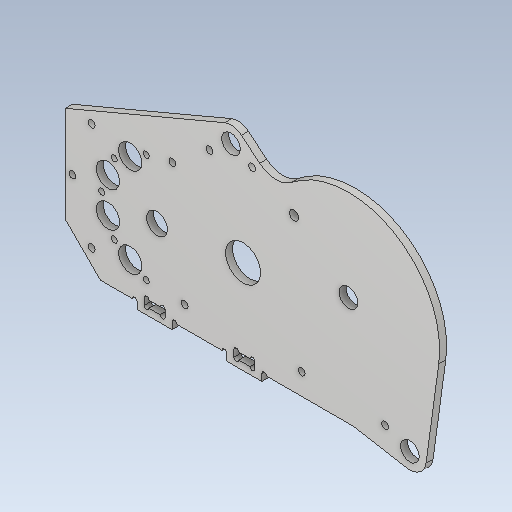
# Autodesk Inventor part: アーム真ん中フレーム
Saved by Autodesk Inventor 2020 (Build 240168000, 168)
## iProperties
Created: 2019-12-03
Part Number: アーム真ん中フレーム
Material: アルミニウム 2014-T4
Document SubType Name: Modeling
Designer: tanjihayato
Density: 2.8 g/cm^3
Appearance: サテン
Mass: 94.056 g
Surface Area: 251.98 cm^2
Volume: 33.5914 cm^3
Author: tanjihayato
Autodesk Inventor part; units mm, degrees
note: some values were not read from the file. Chosen so that the rebuilt part matches the saved one: sketch regions of "押し出し1".
ref_plane "YZ Plane" through (0, 0, 0) normal (1, 0, 0) x (0, 1, 0)
ref_plane "XZ Plane" through (0, 0, 0) normal (0, 1, 0) x (-1, 0, 0)
ref_plane "XY Plane" through (0, 0, 0) normal (0, 0, 1) x (1, 0, 0)
sketch "スケッチ1" plane through (0, 0, 0) normal (0, 0, 1) x (1, 0, 0)
  line L0 (-170.6512, -31.4118) -> (202.8656, -31.4118) construction
  circle A0 centre (-14, -17.4118) radius 14 construction
  circle A1 centre (14, -17.4118) radius 14 construction
  circle A2 centre (-28.0204, 0.0121) radius 20.05 construction
  circle A3 centre (-28.0204, 0.0121) radius 5.05 construction
  circle A4 centre (8.8763, 3.8907) radius 32.05 construction
  circle A5 centre (8.8763, 3.8907) radius 10.1 construction
  circle A6 centre (54.047, 13.5882) radius 36.1 construction
  line L1 (-170.915, -81.4118) -> (490.0044, -81.4118)
  circle A7 centre (-28.0204, 0.0121) radius 22.342 construction
  circle A8 centre (-39.4931, 19.1835) radius 14 construction
  circle A9 centre (-49.0547, 7.5438) radius 14 construction
  circle A10 centre (-49.0547, -7.5196) radius 14 construction
  circle A11 centre (-39.4931, -19.1593) radius 14 construction
  circle A12 centre (8.8763, 3.8907) radius 33.05 construction
  circle A13 centre (54.047, 13.5882) radius 38.1 construction
  line L2 (-11.5565, -29.1593) -> (4.2969, -29.1593) construction
  line L3 (-67.2952, 44.8622) -> (-67.2952, -57.3934) construction
  line L4 (-149.4523, -1.6098) -> (-132.6633, -31.6026)
  line L5 (-132.7701, -31.4118) -> (-132.7701, 74.0456)
  circle A14 centre (-11.4931, -19.1593) radius 14 construction
  line L6 (-197.2268, -33.1593) -> (179.6604, -33.1593) construction
  circle A15 centre (54.047, 13.5882) radius 4.025
  circle A16 centre (54.047, 13.5882) radius 6
  circle A17 centre (-39.4931, 19.1835) radius 5
  circle A18 centre (-49.0547, 7.5438) radius 5
  circle A19 centre (-49.0547, -7.5196) radius 5
  circle A20 centre (-39.4931, -19.1593) radius 5
  circle A21 centre (-39.4931, 19.1835) radius 8 construction
  circle A22 centre (-49.0547, 7.5438) radius 8 construction
  circle A23 centre (-49.0547, -7.5196) radius 8 construction
  circle A24 centre (-39.4931, -19.1593) radius 8 construction
  circle A25 centre (-28.0204, 0.0121) radius 4.5
  circle A26 centre (8.8763, 3.8907) radius 7.5
  line L7 (-17.5497, 32.3149) -> (-46.3578, 15.0755) construction
  line L8 (-46.3578, 15.0755) -> (-51.7515, 0.0121) construction
  line L9 (-51.7515, 0.0121) -> (-46.3578, -15.0513) construction
  line L10 (-46.3578, -15.0513) -> (-37.9391, -20.0892) construction
  circle A27 centre (-32.6283, 23.2915) radius 1.3
  circle A28 centre (-46.3578, 15.0755) radius 1.3
  circle A29 centre (-51.7515, 0.0121) radius 1.3
  circle A30 centre (-46.3578, -15.0513) radius 1.3
  circle A31 centre (-32.6283, -23.2673) radius 1.3
  line L11 (-67.2952, 23.1796) -> (-67.2952, -18.1327)
  arc A32 (79.2003, -37.212) -> (87.3507, -31.2711) centre (80.4159, -30.3183) ccw
  arc A33 (8.1864, 50.8943) -> (0.9804, 51.9708) centre (3.7003, 45.5208) ccw
  line L12 (-52.2685, -33.1593) -> (56.2168, -33.1593)
  line L13 (56.2168, -33.1593) -> (79.2003, -37.212)
  arc A34 (92.7831, 8.2659) -> (29.742, 44.2162) centre (54.047, 13.5882) ccw
  line L14 (87.3507, -31.2711) -> (92.7831, 8.2659)
  line L15 (0.9804, 51.9708) -> (-67.2952, 23.1796)
  circle A35 centre (34.0114, -24.0061) radius 4.5 construction
  circle A36 centre (34.0114, -24.0061) radius 1.5
  circle A37 centre (-21.4477, 26.0369) radius 4.5 construction
  circle A38 centre (-21.4477, 26.0369) radius 1.5
  circle A39 centre (-56.0504, 23.0377) radius 1.5
  circle A40 centre (-56.0504, 23.0377) radius 3 construction
  circle A41 centre (-56.0504, 23.0377) radius 4.5 construction
  circle A42 centre (-64.2952, 0.0121) radius 1.5
  circle A43 centre (-64.2952, 0.0121) radius 3 construction
  circle A44 centre (-64.2952, 0.0121) radius 4.3311 construction
  line L16 (54.047, 13.5882) -> (103.0278, 23.6322)
  line L17 (103.0278, 23.6322) -> (59.4403, 12.4461)
  line L18 (59.4403, 12.4461) -> (30.7326, 32.4678)
  line L19 (30.7326, 32.4678) -> (54.047, 13.5882)
  line L20 (103.0278, 23.6322) -> (519.5307, 130.5215)
  line L21 (-183.2789, 162.2213) -> (-183.2789, -125.2315)
  line L22 (516.7211, 155.5913) -> (516.7211, -155.5644)
  circle A45 centre (103.0278, 23.6322) radius 7.25
  arc A46 (101.805, 33.809) -> (106.8568, 14.1242) centre (103.0278, 23.6322) ccw
  line L23 (141.7723, 33.5754) -> (440.8907, 56.5571) construction
  line L24 (241.9124, 41.2693) -> (202.3713, 99.0317) construction
  circle A47 centre (3.7003, 45.5208) radius 4
  circle A48 centre (127.2431, 29.8467) radius 2
  circle A49 centre (141.7723, 33.5754) radius 2
  arc A50 (143.6401, 28.9373) -> (141.1758, 38.5397) centre (141.7723, 33.5754) ccw
  line L25 (143.6401, 28.9373) -> (106.8568, 14.1242)
  line L26 (141.1758, 38.5397) -> (101.805, 33.809)
  circle A51 centre (30.7326, 32.4678) radius 2
  circle A52 centre (-16.1798, -24.0771) radius 4.5 construction
  circle A53 centre (-16.1798, -24.0771) radius 1.5
  line L27 (-67.2952, -18.1327) -> (-52.2685, -33.1593)
  circle A54 centre (-56.0504, -23.0135) radius 1.5
  circle A55 centre (-56.0504, -23.0135) radius 3 construction
  circle A56 centre (30.7326, 32.4678) radius 4
  arc A57 (55.034, 16.9462) -> (53.2318, 10.1845) centre (54.047, 13.5882) ccw
  line L28 (99.9171, 22.9943) -> (104.0308, 26.6451) construction
  line L29 (104.0308, 26.6451) -> (105.1356, 21.2572) construction
  line L30 (105.1356, 21.2572) -> (99.9171, 22.9943) construction
  circle A58 centre (105.1356, 21.2572) radius 1.5
  circle A59 centre (104.0308, 26.6451) radius 1.5
  circle A60 centre (99.9171, 22.9943) radius 1.5
  circle A61 centre (103.0278, 23.6322) radius 6
  arc A62 (106.7324, 15.9819) -> (96.5933, 29.1862) centre (103.0278, 23.6322) ccw
  arc A63 (55.034, 16.9462) -> (96.5933, 29.1862) centre (66.3134, 55.3229) ccw
  arc A64 (53.2318, 10.1845) -> (106.7324, 15.9819) centre (71.8656, 87.9841) ccw
  circle A65 centre (54.047, 13.5882) radius 8.5
  line L31 (101.3203, 31.9589) -> (52.3395, 21.9149)
  line L32 (55.7545, 5.2615) -> (104.7353, 15.3054)
  circle A66 centre (12.7384, 41.2415) radius 3 construction
  circle A67 centre (12.7384, 41.2415) radius 4.5 construction
  circle A68 centre (12.7384, 41.2415) radius 1.5
  circle A69 centre (80.4159, -30.3183) radius 4
  circle A70 centre (69.7531, -26.0108) radius 1.5
  circle A71 centre (69.7531, -26.0108) radius 4.5 construction
  circle A72 centre (-56.0504, -23.0135) radius 4.5 construction
  line L33 (8.1864, 50.8943) -> (15.9809, 44.3871)
  arc A73 (15.9809, 44.3871) -> (29.742, 44.2162) centre (22.9664, 52.7545) ccw
  circle A74 centre (-5.4761, 38.5895) radius 1.5
  circle A75 centre (-5.4761, 38.5895) radius 4.5 construction
  circle A76 centre (54.047, 13.5882) radius 50 construction
  circle A77 centre (3.7003, 45.5208) radius 2
  circle A78 centre (80.4159, -30.3183) radius 2
  point P0 (0, 0)
  point P1 (0, 0)
  point P2 (-49.0547, 7.5438)
  point P3 (-49.0547, -7.5196)
  dimension "d89" = 100
  dimension "d0" = 40.1
  dimension "d1" = 10.1
  dimension "d2" = 64.1
  dimension "d3" = 20.2
  dimension "d4" = 72.2
  dimension "d5" = 95
  dimension "d6" = 44.684
  dimension "d7" = 28
  dimension "d8" = 28
  dimension "d9" = 28
  dimension "d10" = 28
  dimension "d11" = 1
  dimension "d12" = 2
  dimension "d13" = 4
  dimension "d14" = 8.05
  dimension "d15" = 12
  dimension "d16" = 10
  dimension "d17" = 10
  dimension "d18" = 10
  dimension "d19" = 10
  dimension "d20" = 3
  dimension "d21" = 3
  dimension "d22" = 3
  dimension "d23" = 3
  dimension "d24" = 9
  dimension "d25" = 15
  dimension "d26" = 2.6
  dimension "d27" = 2.6
  dimension "d28" = 2.6
  dimension "d29" = 2.6
  dimension "d30" = 2.6
  dimension "d31" = 1
  dimension "d32" = 9
  dimension "d33" = 3
  dimension "d34" = 9
  dimension "d35" = 3
  dimension "d36" = 3
  dimension "d37" = 6
  dimension "d38" = 9
  dimension "d39" = 3
  dimension "d40" = 6
  dimension "d41" = 50
  dimension "d42" = 45
  dimension "d43" = 35
  dimension "d44" = 30
  dimension "d45" = 39
  dimension "d46" = 430
  dimension "d47" = 700
  dimension "d48" = 14.5
  dimension "d49" = 3
  dimension "d50" = 300
  dimension "d51" = 10
  dimension "d52" = 70
  dimension "d53" = 120
  dimension "d54" = 140
  dimension "d55" = 8
  dimension "d56" = 4
  dimension "d57" = 4
  dimension "d58" = 15
  dimension "d59" = 25
  dimension "d60" = 10
  dimension "d61" = 4
  dimension "d62" = 9
  dimension "d63" = 3
  constraints: 75 centre point, 68 end point, 51 tangent, 41 coincident, 30 point on circle, 13 point on line, 4 midpoint, 4 vertical, 2 collinear, 2 horizontal, 1 vertical alignment, 21 other
  measures "d0" diameter of A2
  measures "d1" diameter of A3
  measures "d2" diameter of A4
  measures "d3" diameter of A5
  measures "d4" diameter of A6
  measures "d5" distance from line of L1 A6.centre
  measures "d6" diameter of A7
  measures "d7" diameter of A8
  measures "d8" diameter of A9
  measures "d9" diameter of A10
  measures "d10" diameter of A11
  measures "d11" radial gap between concentric circles of A4 A12
  measures "d12" radial gap between concentric circles of A6 A13
  measures "d13" distance between parallel lines of L6 L2
  measures "d14" diameter of A15
  measures "d15" diameter of A16
  measures "d16" diameter of A17
  measures "d17" diameter of A18
  measures "d18" diameter of A19
  measures "d19" diameter of A20
  measures "d20" radial gap between concentric circles of A17 A21
  measures "d24" diameter of A25
  measures "d25" diameter of A26
  measures "d26" diameter of A27
  measures "d27" diameter of A28
  measures "d28" diameter of A29
  measures "d29" diameter of A30
  measures "d30" diameter of A31
  measures "d31" radial gap between concentric circles of A13 A34
  measures "d32" diameter of A35
  measures "d33" diameter of A36
  measures "d34" diameter of A37
  measures "d35" diameter of A38
  measures "d36" diameter of A39
  measures "d37" diameter of A40
  measures "d38" diameter of A41
  measures "d39" diameter of A42
  measures "d40" diameter of A43
  measures "d41" distance of L16.start L16.end
  measures "d42" distance of L16.end L17.end
  measures "d43" distance of L17.end L18.end
  measures "d44" distance of L18.end L16.start
  measures "d45" angle of L0 L19
  measures "d46" distance of L16.end L20.end
  measures "d47" distance between parallel lines of L22 L21
  measures "d48" diameter of A45
  measures "d49" radial gap between concentric circles of A45 A46
  measures "d50" distance of L23.start L23.end
  measures "d51" angle of L20 L23
  measures "d52" distance of L24.start L24.end
  measures "d53" angle of L23 L24
  measures "d54" distance of L16.end L24.start
  measures "d55" diameter of A47
  measures "d56" diameter of A48
  measures "d57" diameter of A49
  measures "d58" distance of L23.start A48.centre
  measures "d59" distance of A48.centre A45.centre
  measures "d60" diameter of A50
  measures "d61" diameter of A51
  measures "d62" diameter of A52
  measures "d63" diameter of A53
extrude "押し出し1" add sketch "スケッチ1" along normal blind 3 contours A15 L16 A16 L17 L18 | A15 A63 A16 L16 | L18 L17 A16 A64 A15 | A15 L18 A16 A63 | L16 A65 L17 A16 | A16 A63 A65 L16 | A64 A16 L19 A15 | A15 L19 A16 L18 | A16 L18 A65 A63 | A65 A63 L16 | L16 A63 L17 A65 | A64 A65 L19 A16 | A16 L17 A65 A64 | A16 L19 A65 L18 | A65 L31 A34 A63 L16 | L16 A63 L17 | A65 L17 A63 A34 L32 A64 | A64 L32 A65 | A65 L19 A56 L18 | L18 A56 L19 A65 L32 A64 A34 L14 A32 L13 L12 L27 L11 L15 A33 L33 A73 L31 | A63 A34 L16 | L16 A34 L17 A63 | L17 A63 | L32 A34 A64 | A56 L19 A51 L18 | L18 A51 L19 A56
sketch "スケッチ2" plane through (0, 0, 0) normal (0, 0, -1) x (-1, 0, 0)
  circle A0 centre (-3.7003, 45.5208) radius 4
  circle A1 centre (-80.4159, -30.3183) radius 4
  line L0 (67.2952, 23.1796) -> (67.2952, -18.1327)
  line L1 (-0.9804, 51.9708) -> (67.2952, 23.1796)
  arc A2 (-0.9804, 51.9708) -> (-8.1864, 50.8943) centre (-3.7003, 45.5208) ccw
  line L2 (-15.9809, 44.3871) -> (-8.1864, 50.8943)
  arc A3 (-29.742, 44.2162) -> (-15.9809, 44.3871) centre (-22.9664, 52.7545) ccw
  arc A4 (-29.742, 44.2162) -> (-92.7831, 8.2659) centre (-54.047, 13.5882) ccw
  line L3 (-87.3507, -31.2711) -> (-92.7831, 8.2659)
  arc A5 (-87.3507, -31.2711) -> (-79.2003, -37.212) centre (-80.4159, -30.3183) ccw
  line L4 (-56.2168, -33.1593) -> (-79.2003, -37.212)
  line L5 (52.2685, -33.1593) -> (-56.2168, -33.1593)
  line L6 (67.2952, -18.1327) -> (52.2685, -33.1593)
  circle A6 centre (32.6283, 23.2915) radius 1.3
  circle A7 centre (46.3578, 15.0755) radius 1.3
  circle A8 centre (51.7515, 0.0121) radius 1.3
  circle A9 centre (46.3578, -15.0513) radius 1.3
  circle A10 centre (32.6283, -23.2673) radius 1.3
  circle A11 centre (-34.0114, -24.0061) radius 1.5
  circle A12 centre (21.4477, 26.0369) radius 1.5
  circle A13 centre (56.0504, 23.0377) radius 1.5
  circle A14 centre (64.2952, 0.0121) radius 1.5
  circle A15 centre (16.1798, -24.0771) radius 1.5
  circle A16 centre (56.0504, -23.0135) radius 1.5
  circle A17 centre (-12.7384, 41.2415) radius 1.5
  circle A18 centre (-69.7531, -26.0108) radius 1.5
  circle A19 centre (5.4761, 38.5895) radius 1.5
  circle A20 centre (28.0204, 0.0121) radius 4.5
  circle A21 centre (39.4931, 19.1835) radius 5
  circle A22 centre (49.0547, 7.5438) radius 5
  circle A23 centre (49.0547, -7.5196) radius 5
  circle A24 centre (39.4931, -19.1593) radius 5
  circle A25 centre (-8.8763, 3.8907) radius 7.5
  circle A26 centre (-30.7326, 32.4678) radius 2
  circle A27 centre (-54.047, 13.5882) radius 4.025
  line L7 (-11.0425, -49.8237) -> (-11.0425, -46.8237)
  line L8 (3.9575, -46.8237) -> (3.9575, -49.8237)
  line L9 (27.4427, -49.8237) -> (27.4427, -46.8237)
  circle A28 centre (54.9427, -18.301) radius 5
  line L10 (42.4427, -46.8237) -> (42.4427, -49.8237)
  line L11 (36.5547, -33.1593) -> (36.5547, -36.1593)
  line L12 (36.5547, -36.1593) -> (21.5547, -36.1593)
  line L13 (21.5547, -36.1593) -> (21.5547, -33.1593)
  line L14 (-1.9305, -33.1593) -> (-1.9305, -36.1593)
  line L15 (-1.9305, -36.1593) -> (-16.9305, -36.1593)
  line L16 (-16.9305, -36.1593) -> (-16.9305, -33.1593)
  circle A29 centre (37.6047, -33.1593) radius 1.05
  circle A30 centre (20.5047, -33.1593) radius 1.05
  circle A31 centre (-0.8805, -33.1593) radius 1.05
  circle A32 centre (-17.9805, -33.1593) radius 1.05
  line L17 (-13.9305, -33.1593) -> (-13.9305, -30.1593)
  line L18 (-13.9305, -30.1593) -> (-4.9305, -30.1593)
  line L19 (-4.9305, -30.1593) -> (-4.9305, -33.1593)
  line L20 (52.2685, -33.1593) -> (-56.2168, -33.1593)
  line L21 (24.5547, -33.1593) -> (24.5547, -30.1593)
  line L22 (24.5547, -30.1593) -> (33.5547, -30.1593)
  line L23 (33.5547, -30.1593) -> (33.5547, -33.1593)
  circle A33 centre (-12.8805, -30.1593) radius 1.05
  circle A34 centre (-5.9805, -30.1593) radius 1.05
  circle A35 centre (-12.8805, -33.1593) radius 1.05
  circle A36 centre (-5.9805, -33.1593) radius 1.05
  circle A37 centre (25.6047, -30.1593) radius 1.05
  circle A38 centre (32.5047, -30.1593) radius 1.05
  circle A39 centre (25.6047, -33.1593) radius 1.05
  circle A40 centre (32.5047, -33.1593) radius 1.05
  point P0 (0, 0)
  point P1 (0, 0)
  dimension "d95" = 12.5
  dimension "d96" = 15
  dimension "d97" = 23.4852
  dimension "d98" = 3
  dimension "d99" = 15
  dimension "d100" = 3
  dimension "d101" = 15
  dimension "d102" = 12.5
  dimension "d103" = 23.4852
  dimension "d104" = 2.1
  dimension "d105" = 2.1
  dimension "d106" = 2.1
  dimension "d107" = 2.1
  dimension "d108" = 3
  dimension "d109" = 9
  dimension "d110" = 3
  dimension "d111" = 9
  dimension "d112" = 3
  dimension "d113" = 3
  dimension "d114" = 2.1
  dimension "d115" = 2.1
  dimension "d116" = 2.1
  dimension "d117" = 2.1
  dimension "d118" = 2.1
  dimension "d119" = 2.1
  dimension "d120" = 2.1
  dimension "d121" = 2.1
  constraints: 44 end point, 41 centre point, 12 tangent, 8 point on circle, 6 perpendicular, 5 vertical, 4 point on line, 1 horizontal, 22 other
  measures "d95" distance from line of L10 A28.centre
  measures "d96" distance between parallel lines of L9 L10
  measures "d97" distance between parallel lines of L8 L9
  measures "d98" distance of L11.start L11.end
  measures "d99" distance of L11.end L12.end
  measures "d100" distance of L14.start L14.end
  measures "d101" distance of L14.end L15.end
  measures "d102" distance from line of L11 A23.centre
  measures "d103" distance between parallel lines of L14 L13
  measures "d104" diameter of A29
  measures "d105" diameter of A30
  measures "d106" diameter of A31
  measures "d107" diameter of A32
  measures "d108" distance of L17.start L17.end
  measures "d109" distance of L17.end L18.end
  measures "d110" distance of L21.start L21.end
  measures "d111" distance of L21.end L22.end
  measures "d112" distance between parallel lines of L16 L17
  measures "d113" distance between parallel lines of L11 L23
  measures "d114" diameter of A33
  measures "d115" diameter of A34
  measures "d116" diameter of A35
  measures "d117" diameter of A36
  measures "d118" diameter of A37
  measures "d119" diameter of A38
  measures "d120" diameter of A39
  measures "d121" diameter of A40
extrude "押し出し2" add sketch "スケッチ2" against normal blind 3 contours L11 L12 L13 L5 A39 A40 | A40 L5 | A39 L5 | L14 L15 L16 L5 A35 A36 | A36 L5 | L5 A35 picked at (32.3059, -33.7727) picked at (25.9248, -33.4057) picked at (-5.6407, -33.2431) picked at (-12.5706, -33.322)
extrude "押し出し3" cut sketch "スケッチ2" against normal blind 3 contours A29 L5 | L5 A29 | A40 L5 | A40 L5 A39 L21 A37 L22 A38 L23 | L5 A40 | A38 L22 | L22 A38 | A39 L5 | L5 A39 | A30 L5 | L5 A30 | A37 L22 | L22 A37 | A31 L5 | L5 A31 | A32 L5 | L5 A32 | A36 L5 | A36 L5 A35 L17 A33 L18 A34 L19 | L5 A36 | A35 L5 | L5 A35 | A34 L18 | L18 A34 | A33 L18 | L18 A33
equation "\"d102\" = d95"
equation "\"d103\" = d97"
